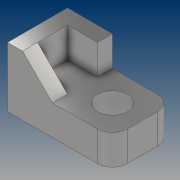
# Autodesk Inventor part: 2
Saved by Autodesk Inventor 2020.2 (Build 242310000, 310)
## iProperties
Created: 2020-09-17
Part Number: 2
Material: 鋼、碳鋼
Document SubType Name: Modeling
Designer: user
Density: 7.85 g/cm^3
Appearance: 半拋光
Mass: 493.438 g
Surface Area: 134.536 cm^2
Volume: 62.8584 cm^3
Author: user
Autodesk Inventor part; units mm, degrees
ref_plane "YZ Plane" through (0, 0, 0) normal (1, 0, 0) x (0, 1, 0)
ref_plane "XZ Plane" through (0, 0, 0) normal (0, 1, 0) x (-1, 0, 0)
ref_plane "XY Plane" through (0, 0, 0) normal (0, 0, 1) x (1, 0, 0)
sketch "草圖1" plane through (0, 0, 0) normal (0, 1, 0) x (-1, 0, 0)
  line L0 (50, -20) -> (-20, -20)
  line L1 (-20, -20) -> (-20, 20)
  line L2 (-20, 20) -> (50, 20)
  line L3 (50, 20) -> (50, -20)
  point P0 (0, 0)
  dimension "d0" = 20
  dimension "d1" = 40
  dimension "d2" = 20
  dimension "d3" = 70
  constraints: 8 end point, 2 parallel, 1 horizontal, 1 perpendicular
  measures "d0" distance from line of L1 point (0, 0)
  measures "d1" distance of L0.end L1.end
  measures "d2" distance from line of point (0, 0) L0
  measures "d3" distance of L0.start L0.end
extrude "擠出1" add sketch "草圖1" along normal blind 40
sketch "草圖2" plane through (-50, 0, 20) normal (0, 0, 1) x (1, 0, 0)
  line L0 (0, 0) -> (0, 40) projected
  line L1 (0, 40) -> (70, 40) projected
  line L2 (70, 40) -> (70, 0) projected
  line L3 (70, 0) -> (0, 0) projected
  line L4 (70, 0) -> (70, 40) projected
  line L5 (70, 40) -> (30, 40)
  line L6 (30, 40) -> (30, 20)
  line L7 (30, 20) -> (70, 20)
  line L8 (70, 20) -> (70, 40)
  point P0 (50, 0)
  point P1 (30, 40)
  dimension "d6" = 40
  dimension "d7" = 20
  constraints: 8 end point, 2 parallel, 1 horizontal, 1 perpendicular
  measures "d6" distance between parallel lines of L2 L6
  measures "d7" distance of L5.end L6.end
extrude "擠出2" cut sketch "草圖2" against normal through all contours L1 L2 L7 L6
sketch "草圖3" plane through (0, 0, 0) normal (0, 0, 1) x (1, 0, 0)
  line L0 (-20, 40) -> (-20, 20) projected
  line L1 (-20, 20) -> (20, 20) projected
  line L2 (20, 20) -> (20, 0) projected
  line L3 (20, 0) -> (-50, 0) projected
  line L4 (-50, 0) -> (-50, 40) projected
  line L5 (-50, 40) -> (-20, 40) projected
  line L6 (-40, 42.2655) -> (11.1327, 42.2655)
  line L7 (11.1327, 42.2655) -> (11.1327, 20)
  line L8 (11.1327, 20) -> (-40, 20)
  line L9 (-40, 20) -> (-40, 42.2655)
  point P0 (0, 0)
  point P1 (-20, 20)
  dimension "d10" = 10
  constraints: 8 end point, 2 parallel, 1 collinear, 1 horizontal, 1 perpendicular
  measures "d10" distance between parallel lines of L9 L4
extrude "擠出3" cut sketch "草圖3" along normal mid plane 20 contours L5 L9 L6 L7 L1 L0 | L0 L8 L9 L5
sketch "草圖4" plane through (-50, 0, 20) normal (0, 0, 1) x (1, 0, 0)
  line L0 (0, 40) -> (30, 40) projected
  line L1 (30, 40) -> (30, 20) projected
  line L2 (30, 20) -> (70, 20) projected
  line L3 (70, 20) -> (70, 0) projected
  line L4 (70, 0) -> (0, 0) projected
  line L5 (0, 0) -> (0, 40) projected
  line L6 (30, 20) -> (70, 20) projected
  line L7 (10, 40) -> (10, 20) projected
  line L8 (30, 20) -> (10, 40)
  point P0 (50, 0)
  constraints: 2 end point
extrude "擠出4" cut sketch "草圖4" against normal blind 17.25 contours L0 L1 L8
sketch "草圖5" plane through (-20, 20, -20) normal (0, 1, 0) x (1, 0, 0)
  line L0 (-20, -10) -> (-20, -30) projected
  line L1 (-20, -30) -> (0, -30) projected
  line L2 (0, -30) -> (0, -40) projected
  line L3 (40, -40) -> (0, -40) projected
  line L4 (40, 0) -> (40, -40) projected
  line L5 (0, 0) -> (40, 0) projected
  line L6 (-30, 0) -> (0, 0) projected
  line L7 (-30, -40) -> (-30, 0) projected
  line L8 (0, -40) -> (-30, -40) projected
  line L9 (0, -10) -> (-20, -10) projected
  line L10 (0, 0) -> (0, -10) projected
  circle A0 centre (20, -20) radius 10
  dimension "d15" = 20
  constraints: 1 centre point, 1 coincident
  measures "d15" diameter of A0
extrude "擠出5" cut sketch "草圖5" against normal through all contours A0
fillet "圓角1" radius 10 2 edges at (20, 10, 20) (20, 10, -20)
